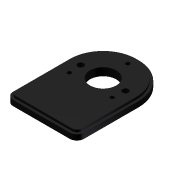
# Autodesk Inventor part: HEDS-5500_A
Saved by Autodesk Inventor 2011 SP1 (Build 150282100, 282)
## iProperties
Created: 2012-12-12
Part Number: HEDS-5500_A
Document SubType Name: Modeling
Designer: arihon
Density: 1 g/cm^3
Author: arihon
Autodesk Inventor part; units mm, degrees
ref_plane "YZ Plane" through (0, 0, 0) normal (1, 0, 0) x (0, 1, 0)
ref_plane "XZ Plane" through (0, 0, 0) normal (0, 1, 0) x (-1, 0, 0)
ref_plane "XY Plane" through (0, 0, 0) normal (0, 0, 1) x (1, 0, 0)
sketch "スケッチ1" plane through (0, 0, 0) normal (0, 0, 1) x (1, 0, 0)
  line L0 (-15, 0.0806) -> (15, 0.0806)
  line L1 (15, 0.0806) -> (15, -26.1194)
  line L2 (15, -26.1194) -> (-15, -26.1194)
  line L3 (-15, -26.1194) -> (-15, 0.0806)
  circle A0 centre (0, 0) radius 15.0002
  dimension "d0" = 30
  dimension "d1" = 15
  dimension "d2" = 26.2
  constraints: 8 end point, 2 parallel, 1 coincident, 1 horizontal, 1 perpendicular, 3 other
  measures "d0" distance of L1.end L2.end
  measures "d1" distance from line of L3 point (0, 0)
  measures "d2" distance of L2.end L0.start
extrude "押し出し1" add sketch "スケッチ1" along normal blind 3.3
sketch "スケッチ2" plane through (0, 0, 3.3) normal (0, 0, 1) x (1, 0, 0)
  arc A0 (15, -0.0806) -> (-15, -0.0806) centre (0, 0) ccw projected
  circle A1 centre (0, 0) radius 9.5
  point P0 (-9.5, 0)
  point P1 (9.5, 0)
  dimension "d5" = 19
  constraints: 2 point on circle, 1 centre point, 1 coincident
  measures "d5" diameter of A1
hole "Hole1" at (-9.5, 0, 3.3) at (9.5, 0, 3.3) direction (0, 0, -1) diameter 2.6 depth 10
sketch "スケッチ3" plane through (0, 0, 3.3) normal (0, 0, 1) x (1, 0, 0)
  arc A0 (15, -0.0806) -> (-15, -0.0806) centre (0, 0) ccw projected
  constraints: 1 coincident
hole "Hole2" at (0, 0, 3.3) direction (0, 0, -1) diameter 11.1 depth 10 tip angle 118
sketch "スケッチ4" plane through (0, 0, 3.3) normal (0, 0, 1) x (1, 0, 0)
  arc A0 (15, -0.0806) -> (-15, -0.0806) centre (0, 0) ccw projected
  line L0 (-15, -26.1194) -> (-15, -0.0806) projected
  line L1 (15, -26.1194) -> (-15, -26.1194) projected
  line L2 (15, -0.0806) -> (15, -26.1194) projected
  line L3 (-14, -0.0806) -> (14, -0.0806)
  line L4 (14, -0.0806) -> (14, -25.1194)
  line L5 (14, -25.1194) -> (-14, -25.1194)
  line L6 (-14, -25.1194) -> (-14, -0.0806)
  circle A1 centre (0, 0) radius 14.0002
  dimension "d20" = 1
  dimension "d21" = 1
  dimension "d22" = 1
  constraints: 8 end point, 2 parallel, 1 coincident, 1 horizontal, 1 perpendicular, 3 other
  measures "d20" distance between parallel lines of L0 L6
  measures "d21" distance between parallel lines of L2 L4
  measures "d22" distance between parallel lines of L1 L5
extrude "押し出し2" cut sketch "スケッチ4" against normal blind 1
fillet "フィレット1" radius 3 2 edges at (15, -26.1194, 1.15) (-15, -26.1194, 1.15)
fillet "フィレット2" radius 2 2 edges at (14, -25.1194, 2.8) (-14, -25.1194, 2.8)
sketch "スケッチ5" plane through (0, 0, 3.3) normal (0, 0, 1) x (1, 0, 0)
  circle A0 centre (0, 0) radius 5.55 projected
  circle A1 centre (0, 0) radius 10.45
  point P0 (0, 10.45)
  point P1 (-9.05, -5.225)
  point P2 (9.05, -5.225)
  dimension "d27" = 20.9
  dimension "d30" = 360
  constraints: 1 coincident, 1 vertical alignment, 6 other
hole "Hole3" at (0, 10.45, 3.3) at (-9.05, -5.225, 3.3) at (9.05, -5.225, 3.3) direction (0, 0, -1) diameter 1.7 end through all
equation "\"d1\" = 0.5 * d0"
equation "\"d22\" = d21"
